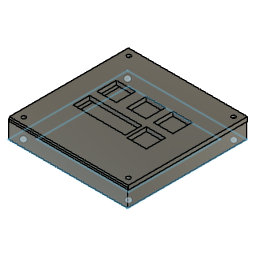
phonographCasing (Autodesk Fusion 360 design; units mm, degrees)
Autodesk Fusion 360 part; units mm, degrees
sketch "Sketch1" plane through (0, 0, 0) normal (0, 0, 1) x (1, 0, 0)
  line L0 (0, 0, -13) -> (66.675, 0, -13)
  line L1 (66.675, 0, -13) -> (66.675, 66.675, -13)
  line L2 (66.675, 66.675, -13) -> (0, 66.675, -13)
  line L3 (0, 66.675, -13) -> (0, 0, -13)
  line L4 (-10.3399, 76.2574, -13) -> (76.3351, 76.2574, -13)
  line L5 (76.3351, 76.2574, -13) -> (76.3351, -10.4176, -13)
  line L6 (76.3351, -10.4176, -13) -> (-10.3399, -10.4176, -13)
  line L7 (-10.3399, -10.4176, -13) -> (-10.3399, 76.2574, -13)
  circle A0 through (-3.545, -5, -13) (-5.7275, -3.7399, -13) (-5.7275, -6.2601, -13)
  circle A1 through (-3.8899, 71.2574, -13) (-6.0649, 72.5131, -13) (-6.0649, 70.0016, -13)
  circle A2 through (73.1009, -5, -13) (70.9259, -3.7443, -13) (70.9259, -6.2557, -13)
  circle A3 through (73.4807, 71.2574, -13) (71.3057, 72.5131, -13) (71.3057, 70.0016, -13)
  dimension "d1" = 66.675
  dimension "d2" = 66.675
  dimension "d3" = 86.675
  dimension "d4" = 86.675
  dimension "d5" = 2.91
  dimension "d6" = 2.9
  dimension "d7" = 2.9
  dimension "d8" = 2.9
extrude "Extrude1" add sketch "Sketch1" along normal blind 3 contours L0 L1 L2 L3 in plane through (0, 0, -13) normal (0, 0, 1) makes body 1
extrude "Extrude2" add sketch "Sketch1" along normal blind 13 contours L4 L5 L6 L7 in plane through (0, 0, -13) normal (0, 0, 1) bodies 1
sketch "Sketch2" plane through (0, 0, 0) normal (0, 0, 1) x (1, 0, 0)
  line L0 (-48.4333, 105.3395) -> (-135.1083, 105.3395)
  line L1 (-135.1083, 105.3395) -> (-135.1083, 18.6645)
  line L2 (-135.1083, 18.6645) -> (-48.4333, 18.6645)
  line L3 (-48.4333, 18.6645) -> (-48.4333, 105.3395)
  line L4 (-97.9431, 81.0654) -> (-83.9431, 81.0654)
  line L5 (-83.9431, 81.0654) -> (-83.9431, 67.0654)
  line L6 (-83.9431, 67.0654) -> (-97.9431, 67.0654)
  line L7 (-97.9431, 67.0654) -> (-97.9431, 81.0654)
  line L8 (-78.8931, 81.5153) -> (-64.8931, 81.5153)
  line L9 (-64.8931, 81.5153) -> (-64.8931, 67.5153)
  line L10 (-64.8931, 67.5153) -> (-78.8931, 67.5153)
  line L11 (-78.8931, 67.5153) -> (-78.8931, 81.5153)
  line L12 (-78.8931, 62.1723) -> (-64.8931, 62.1723)
  line L13 (-64.8931, 62.1723) -> (-64.8931, 48.1723)
  line L14 (-64.8931, 48.1723) -> (-78.8931, 48.1723)
  line L15 (-78.8931, 48.1723) -> (-78.8931, 62.1723)
  line L16 (-119.2264, 61.2342) -> (-81.2264, 61.2342)
  line L17 (-81.2264, 61.2342) -> (-81.2264, 49.2342)
  line L18 (-81.2264, 49.2342) -> (-119.2264, 49.2342)
  line L19 (-119.2264, 49.2342) -> (-119.2264, 61.2342)
  line L20 (-119.0824, 80.5284) -> (-105.0824, 80.5284)
  line L21 (-105.0824, 80.5284) -> (-105.0824, 66.5284)
  line L22 (-105.0824, 66.5284) -> (-119.0824, 66.5284)
  line L23 (-119.0824, 66.5284) -> (-119.0824, 80.5284)
  circle A0 centre (-129.9541, 100.4922) radius 1.45
  circle A1 centre (-53.3828, 100.202) radius 1.45
  circle A2 centre (-129.5, 23.5) radius 1.45
  circle A3 centre (-53.1801, 23.3906) radius 1.45
  dimension "d13" = 86.675
  dimension "d14" = 86.675
  dimension "d17" = 14
  dimension "d18" = 14
  dimension "d19" = 14
  dimension "d20" = 14
  dimension "d21" = 14
  dimension "d22" = 14
  dimension "d23" = 38
  dimension "d24" = 12
  dimension "d25" = 14
  dimension "d26" = 14
  dimension "d27" = 2.9
  dimension "d28" = 2.9
  dimension "d29" = 2.9
  dimension "d30" = 2.9
  constraint horizontal L0
  constraint vertical L1
  constraint horizontal L2
  constraint vertical L3
  constraint horizontal L4
  constraint vertical L5
  constraint horizontal L6
  constraint vertical L7
  constraint horizontal L8
  constraint vertical L9
  constraint horizontal L10
  constraint vertical L11
  constraint horizontal L12
  constraint vertical L13
  constraint horizontal L14
  constraint vertical L15
  constraint horizontal L16
  constraint vertical L17
  constraint horizontal L18
  constraint vertical L19
  constraint horizontal L20
  constraint vertical L21
  constraint horizontal L22
  constraint vertical L23
  measures "d13" distance of L0.start L0.end
  measures "d14" distance of L0.start L2.end
  measures "d17" distance of L4.start L4.end
  measures "d18" distance of L4.end L5.end
  measures "d19" distance of L8.start L8.end
  measures "d20" distance of L8.end L9.end
  measures "d21" distance of L12.start L12.end
  measures "d22" distance of L12.start L14.end
  measures "d23" distance of L16.start L16.end
  measures "d24" distance of L16.start L18.end
  measures "d25" distance of L20.start L20.end
  measures "d26" distance of L20.start L22.end
  measures "d27" diameter of A0
  measures "d28" diameter of A1
  measures "d29" diameter of A2
  measures "d30" diameter of A3
extrude "Extrude3" add sketch "Sketch2" along normal blind 3 separate body makes body 2
move_body "Move1" bodies 2 to x (1, 0, 0) y (0, 1, 0) z (0, 0, 1) at (125.3981, -29.0966, -36.3799)
move_body "Move2" bodies 2 to x (1, 0, 0) y (0, 1, 0) z (0, 0, 1) at (0, 0, 35)
sketch "Sketch3" plane through (-10.3399, 0, 0) normal (-1, 0, 0) x (0, -1, 0)
  line L0 (-76.2574, -13) -> (10.4176, -13)
  line L1 (10.4176, -13) -> (10.4176, 0)
  line L2 (10.4176, 0) -> (-76.2574, 0)
  line L3 (-76.2574, 0) -> (-76.2574, -13)
  line L4 (-44.4535, -0.8387) -> (-34.4535, -0.8387)
  line L5 (-34.4535, -0.8387) -> (-34.4535, -6.8387)
  line L6 (-34.4535, -6.8387) -> (-44.4535, -6.8387)
  line L7 (-44.4535, -6.8387) -> (-44.4535, -0.8387)
  dimension "d33" = 10
  dimension "d34" = 6
  constraint horizontal L4
  constraint vertical L5
  constraint horizontal L6
  constraint vertical L7
  measures "d33" distance of L4.start L4.end
  measures "d34" distance of L4.end L5.end
extrude "Extrude4" cut sketch "Sketch3" against normal blind 13 contours L4 L5 L6 L7 bodies 1
